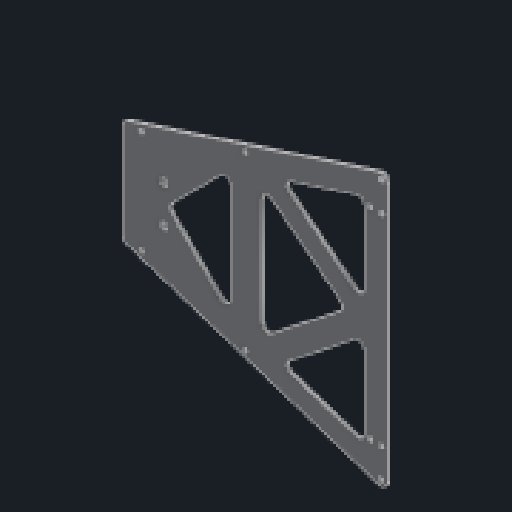
# Autodesk Inventor part: Part1
Saved by Autodesk Inventor 2025.2 (Build 292293000, 293)
## iProperties
Created: 2025-09-26
Part Number: Part1
Material: Generic
Document SubType Name: Sheet Metal
Designer: valer
Density: 1 g/cm^3
Sheet Metal Rule: Default
Appearance: Default
Author: valer
Autodesk Inventor part; units mm, degrees
ref_plane "YZ Plane" through (0, 0, 0) normal (1, 0, 0) x (0, 1, 0)
ref_plane "XZ Plane" through (0, 0, 0) normal (0, 1, 0) x (-1, 0, 0)
ref_plane "XY Plane" through (0, 0, 0) normal (0, 0, 1) x (1, 0, 0)
sketch "Base" plane through (0, 0, 0) normal (0, 0, 1) x (1, 0, 0)
  line L0 (-173.8499, -66.2658) -> (171.6188, -178.9186) construction
  line L1 (-9.525, -101.5493) -> (-9.525, 101.5493) construction
  line L2 (-9.525, 0) -> (-9.525, -119.85)
  line L3 (187.0398, -183.9472) -> (-9.525, -119.85)
  line L4 (187.0398, -183.9472) -> (187.0398, 0)
  line L5 (187.0398, 0) -> (-9.525, 0) construction
  line L6 (-9.525, 0) -> (-9.525, 119.85)
  line L7 (187.0398, 183.9472) -> (-9.525, 119.85)
  line L8 (187.0398, 183.9472) -> (187.0398, 0)
  point P0 (0, 0)
  point P1 (187.0398, -182.4643)
extrude "Plate1" add sketch "Base" along normal blind 3.048
sketch "MountHoles" plane through (0, 0, 0) normal (0, 0, -1) x (-1, 0, 0)
  line L0 (-179.0398, 172.9239) -> (1.525, 114.0441) construction
  circle A0 centre (-179.0398, 172.9239) radius 3
  circle A1 centre (1.525, 114.0441) radius 3
  line L1 (-228.9265, 0) -> (50.7072, 0) construction
  circle A2 centre (-179.0398, -172.9239) radius 3
  circle A3 centre (1.525, -114.0441) radius 3
  line L2 (-187.0398, 183.9472) -> (9.525, 119.85) projected
  point P0 (0, 0)
  dimension "d2" = 6
  dimension "d3" = 6
  dimension "d45" = 8
  constraints: 4 centre point, 2 coincident, 2 end point, 2 symmetric about line, 2 other
  measures "d2" diameter of A0
  measures "d3" diameter of A1
  measures "d45" distance between parallel lines of L2 L0
extrude "MountHolesFeature" cut sketch "MountHoles" against normal blind 3.048
sketch "MiddleCuts" plane through (0, 0, 3.048) normal (0, 0, 1) x (1, 0, 0)
  line L0 (20.475, -87.6609) -> (132.6758, 0)
  line L1 (132.6758, 0) -> (20.475, 87.6609)
  line L2 (20.475, 87.6609) -> (20.475, -87.6609)
  line L3 (157.0398, 19.0353) -> (45.4472, 106.221)
  line L4 (45.4472, 106.221) -> (157.0398, 142.6099)
  line L5 (157.0398, 142.6099) -> (157.0398, 19.0353)
  line L6 (-48.838, 0) -> (226.3528, 0) construction
  line L7 (-9.525, -119.85) -> (-9.525, 119.85) projected
  line L8 (-9.525, 119.85) -> (187.0398, 183.9472) projected
  line L9 (187.0398, 183.9472) -> (187.0398, -183.9472) projected
  line L10 (157.0398, -19.0353) -> (45.4472, -106.221)
  line L11 (45.4472, -106.221) -> (157.0398, -142.6099)
  line L12 (157.0398, -142.6099) -> (157.0398, -19.0353)
  point P0 (0, 0)
  point P1 (-9.525, -114.0441)
  point P2 (-9.525, 114.0441)
  point P3 (-4.0052, 121.6499)
  point P4 (176.5597, 180.5298)
  point P5 (187.0398, 172.9239)
  point P6 (187.0398, -172.9239)
  dimension "d18" = 30
  dimension "d19" = 30
  dimension "d20" = 30
  dimension "d21" = 30
  dimension "d22" = 38
  constraints: 18 end point, 4 parallel, 3 symmetric about line, 2 point on line, 1 equal length, 1 perpendicular
  measures "d18" distance between parallel lines of L7 L2
  measures "d19" distance between parallel lines of L8 L4
  measures "d20" distance between parallel lines of L3 L1
  measures "d21" distance between parallel lines of L9 L5
  measures "d22" angle of L1 L6
extrude "MiddleCutsFeature" cut sketch "MiddleCuts" against normal blind 3.048
fillet "InsideFilletsFeature" radius 8 9 edges at (20.475, -87.6609, 1.524) (20.475, 87.6609, 1.524) (45.4472, 106.221, 1.524) (45.4472, -106.221, 1.524) (157.0398, -142.6099, 1.524) (157.0398, -19.0353, 1.524) (132.6758, 0, 1.524) (157.0398, 19.0353, 1.524) (157.0398, 142.6099, 1.524)
sketch "TorsoLiftMountHoles" plane through (0, 0, 3.048) normal (0, 0, 1) x (1, 0, 0)
  circle A0 centre (180.0398, -133.6037) radius 3 projected
  circle A1 centre (164.0398, -133.6037) radius 3 projected
  circle A2 centre (180.0398, 133.6037) radius 3 projected
  circle A3 centre (164.0398, 133.6037) radius 3 projected
  point P0 (0, 0)
extrude "TorsoLiftMountHolesFeature" cut sketch "TorsoLiftMountHoles" against normal blind 3.048
sketch "Continuation" plane through (0, 0, 0) normal (0, 0, -1) x (-1, 0, 0)
  line L0 (9.525, 119.85) -> (164.525, 69.3065)
  line L1 (-256.7865, 0) -> (231.44, 0) construction
  line L2 (9.525, -119.85) -> (164.525, -69.3065)
  line L3 (164.525, 69.3065) -> (164.525, -69.3065)
  line L4 (-187.0398, 183.9472) -> (9.525, 119.85)
  line L5 (9.525, 119.85) -> (9.525, -119.85)
  circle A0 centre (1.525, 114.0441) radius 3
  line L6 (1.525, 114.0441) -> (164.525, 60.8919) construction
  circle A1 centre (139.525, 69.0441) radius 3
  circle A2 centre (139.525, -69.0441) radius 3
  point P0 (0, 0)
  dimension "d46" = 155
  dimension "d47" = 25
  measures "d46" distance between parallel lines of L5 L3
  measures "d47" distance from line of L3 A1.centre
sheet face with bend "ContinuationFeature" sketch "Continuation" thickness 3.048 toward (0, 0, 1) bend radius 3.048 relief straight relief width 3.048 relief depth 1.524 contours L0 L3 L2 L5
bend "Bend2"
fillet "OutsideFilletsFeature" radius 8 4 edges at (187.0398, -183.9472, 1.524) (187.0398, 183.9472, 1.524) (-164.525, 69.3065, 1.524) (-164.525, -69.3065, 1.524)
sketch "HingeMountHoles" plane through (0, 0, 3.048) normal (0, 0, 1) x (1, 0, 0)
  line L0 (-109.525, -25.4) -> (-109.525, 25.4) construction
  circle A0 centre (-109.525, -25.4) radius 4.7625
  circle A1 centre (-109.525, 25.4) radius 4.7625
  line L1 (-240.838, 0) -> (258.3528, 0) construction
  line L2 (-164.525, -63.5006) -> (-164.525, 63.5006) projected
  point P0 (0, 0)
  point P1 (-109.525, 0)
  dimension "d54" = 9.525
  dimension "d55" = 50.8
  dimension "d56" = 55
  constraints: 2 centre point, 2 coincident, 2 end point, 1 equal radius, 1 midpoint, 1 point on line, 1 vertical
  measures "d54" diameter of A0
  measures "d55" distance of L0.start L0.end
  measures "d56" distance between parallel lines of L2 L0
extrude "Cut5" cut sketch "HingeMountHoles" against normal blind 3.048
sketch "Sketch9" plane through (0, 0, 0) normal (0, 0, -1) x (-1, 0, 0)
  line L0 (20.475, -84.7246) -> (20.475, 84.7246)
  line L1 (20.475, 84.7246) -> (105.1996, 0)
  line L2 (105.1996, 0) -> (20.475, -84.7246)
  line L3 (234.838, 0) -> (-257.3528, 0) construction
  line L4 (-20.475, 71.2585) -> (-20.475, -71.2585) projected
  arc A0 (-59.7335, -110.8796) -> (-57.2884, -96.9697) centre (-62.2137, -103.2737) ccw projected
  line L5 (-59.7335, -110.8796) -> (164.525, -37.7518) construction
  line L6 (164.525, -63.5006) -> (164.525, 63.5006) projected
  line L7 (-59.7335, -110.8796) -> (-146.5597, -139.1925) projected
  point P0 (0, 0)
  point P1 (20.475, 0)
  dimension "d59" = 20.475
  dimension "d60" = 20.475
  dimension "d61" = 45
  constraints: 8 end point, 3 point on line, 1 collinear, 1 midpoint, 1 perpendicular, 1 tangent, 1 vertical
  measures "d59" distance from line of point (0, 0) L4
  measures "d60" distance from line of point (0, 0) L0
  measures "d61" angle of L0 L2
extrude "Cut6" cut sketch "Sketch9" against normal blind 3.048
fillet "Fillet4" radius 8 3 edges at (-20.475, -84.7246, 1.524) (-20.475, 84.7246, 1.524) (-105.1996, 0, 1.524)
equation "\"d7\" = Thickness"
equation "\"d19\" = d18"
equation "\"d23\" = Thickness"
equation "\"d43\" = Thickness"
equation "\"d57\" = Thickness"
equation "\"d60\" = d59"
equation "\"d62\" = Thickness"
equation "\"d0\" = Thickness"
equation "\"d48\" = BendRadius"
equation "\"d49\" = BendReliefWidth"
equation "\"d51\" = MinimumRemnant"
equation "\"d50\" = BendReliefDepth"
equation "\"d52\" = TransitionRadius"
equation "\"BendRadius\" = Thickness"
equation "\"BendReliefWidth\" = Thickness"
equation "\"BendReliefDepth\" = 0.5 * Thickness"
equation "\"CornerReliefSize\" = 4 * Thickness"
equation "\"MinimumRemnant\" = 2 * Thickness"
equation "\"TransitionRadius\" = BendRadius"
equation "\"JacobiRadiusSize\" = BendRadius"
equation "\"GapSize\" = Thickness"
equation "\"Thickness\" = 3.048"
body "Solid1"
